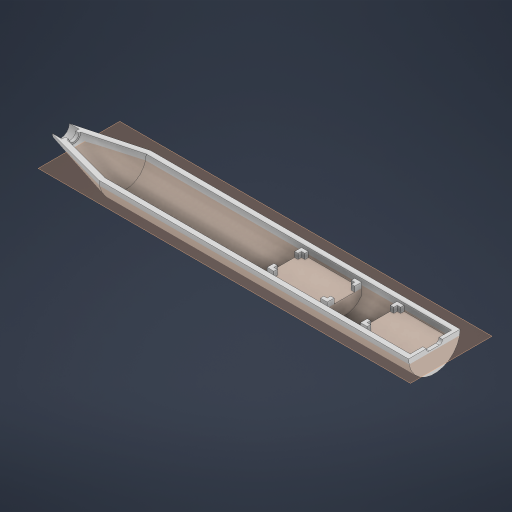
# Autodesk Inventor part: Half bottom
Saved by Autodesk Inventor 2023 (Build 270158000, 158)
## iProperties
Created: 2023-12-06
Part Number: Half bottom
Material: Generic
Document SubType Name: Modeling
Designer: Andi
Density: 1 g/cm^3
Appearance: Default
Author: Andi
Autodesk Inventor part; units mm, degrees
ref_plane "YZ Plane" through (0, 0, 0) normal (1, 0, 0) x (0, 1, 0)
ref_plane "XY Plane" through (0, 0, 0) normal (0, 0, 1) x (1, 0, 0)
sketch "Sketch1" plane through (0, 0, 0) normal (0, 1, 0) x (-1, 0, 0)
  line L0 (90, -15) -> (-90, -15)
  line L1 (-90, -15) -> (-90, 0)
  line L2 (-90, 15) -> (90, 15) construction
  line L3 (90, -15) -> (127.3205, -5)
  line L4 (145.9808, 0) -> (127.3205, 5) construction
  line L5 (127.3205, -5) -> (145.9808, 0) construction
  line L6 (127.3205, 5) -> (90, 15) construction
  line L7 (145.9808, 0) -> (-90, 0)
  line L8 (-88, -12) -> (89.605, -12)
  line L9 (89.605, -12) -> (119.6622, -3.9462)
  line L10 (-90, 0) -> (-88, 0)
  line L11 (-88, 0) -> (-88, -12)
  line L12 (-90, 0) -> (-90, 15) construction
  arc A0 (126.6622, -5) -> (126.6622, 5) centre (126.6622, 0) ccw construction
  line L13 (126.6622, -5) -> (121.6622, -5) construction
  line L14 (121.6622, -5) -> (121.6622, 5) construction
  line L15 (121.6622, 5) -> (126.6622, 5) construction
  line L16 (90, -15) -> (90, 15) construction
  line L17 (119.6622, -3.9462) -> (119.6622, -3)
  line L18 (119.6622, -3) -> (121.6622, -3)
  line L19 (121.6622, -3) -> (121.6622, -5)
  line L20 (121.6622, -5) -> (127.3205, -5)
  point P0 (0, 0)
  point P1 (-88, 0)
  point P2 (131.6622, 0)
  point P3 (90, 0)
  dimension "d0" = 180
  dimension "d1" = 30
  dimension "d2" = 3
  dimension "d3" = 2
  dimension "d5" = 30
  dimension "d6" = 90
  dimension "d9" = 3
  dimension "d24" = 10
  dimension "d25" = 10
  dimension "d26" = 2
  dimension "d29" = 2
  constraints: 43 end point, 8 perpendicular, 3 horizontal, 3 point on circle, 3 tangent, 2 collinear, 2 equal length, 2 horizontal alignment, 2 parallel, 2 point on line, 2 vertical, 1 centre point, 1 midpoint
  measures "d0" distance of L2.start L2.end
  measures "d1" distance of L0.end L2.start
  measures "d2" distance between parallel lines of L8 L0
  measures "d3" distance between parallel lines of L11 L1
  measures "d5" angle of L4 L5
  measures "d6" distance from line of point (0, 0) L1
  measures "d9" distance between parallel lines of L9 L3
  measures "d24" diameter of A0
  measures "d25" distance from line of point (131.662, 0) L14
  measures "d26" distance of L17.end L18.end
  measures "d29" distance of L18.end L13.end
revolve "Revolution1" add sketch "Sketch1" angle 180 about axis through (-145.9808, 0, 0) along (-1, 0, 0)
ref_plane "Work Plane1" through (0, -3, 0) normal (0, 1, 0) x (-1, 0, 0)
sketch "Sketch2" plane through (0, -3, 0) normal (0, 1, 0) x (-1, 0, 0)
  line L0 (-57.7, -10.7) -> (-88, -10.7)
  line L1 (-88, -10.7) -> (-88, 10.7)
  line L2 (-88, 10.7) -> (-57.7, 10.7)
  line L3 (-57.7, 10.7) -> (-57.7, -10.7)
  line L4 (-88, -12) -> (-88, 12) construction
  line L5 (-88, -12) -> (-88, 12) construction
  line L6 (-2.7, -10) -> (-37.7, -10)
  line L7 (-37.7, -10) -> (-37.7, 10)
  line L8 (-37.7, 10) -> (-2.7, 10)
  line L9 (-2.7, 10) -> (-2.7, -10)
  line L10 (17.6, 0) -> (-105.6, 0) construction
  point P0 (0, 0)
  point P1 (-88, 0)
  point P2 (-57.7, 0)
  point P3 (-37.7, 0)
  point P4 (-88, 0)
  point P5 (-88, 0)
  point P6 (-88, 0)
  point P7 (-88, 0)
  point P8 (-59.7, -8.7)
  point P9 (-59.7, 8.7)
  dimension "d20" = 35
  dimension "d21" = 20
  dimension "d39" = 20
  dimension "d42" = 2
  dimension "d43" = 2
  constraints: 16 end point, 7 midpoint, 4 parallel, 2 horizontal, 2 horizontal alignment, 2 perpendicular, 1 point on line, 2 other
  measures "d20" distance of L6.start L6.end
  measures "d21" distance of L8.end L6.start
  measures "d39" distance between parallel lines of L7 L3
  measures "d42" distance from line of point (-59.7, -8.7) L0
  measures "d43" distance from line of L3 point (-59.7, -8.7)
sketch "Sketch3" plane through (90, 0, 15) normal (1, 0, 0) x (0, 0, -1)
  arc A0 (17.89, -1.5) -> (17.89, 1.14) centre (17.89, -0.18) ccw construction
  arc A1 (12.11, 1.14) -> (12.11, -1.5) centre (12.11, -0.18) ccw construction
  line L0 (17.89, -0.18) -> (12.11, -0.18) construction
  line L1 (17.89, -2) -> (12.11, -2)
  line L2 (12.11, 1.64) -> (17.89, 1.64)
  arc A2 (17.89, -2) -> (17.89, 1.64) centre (17.89, -0.18) ccw
  arc A3 (12.11, 1.64) -> (12.11, -2) centre (12.11, -0.18) ccw
  point P0 (15, 0)
  point P1 (15, -0.18)
  dimension "d44" = 0.5
  constraints: 8 end point, 4 point on circle, 4 tangent, 2 centre point, 1 horizontal, 1 midpoint, 1 parallel
  measures "d44" radial gap between concentric circles of A0 A2
extrude "Extrusion2" cut sketch "Sketch3" against normal blind 10
extrude "Extrusion3" add sketch "Sketch2" against normal up to surface round surface about axis through (-0.8025, 0, 0) along (-1, 0, 0) radius 12 far side no
sketch "Sketch4" plane through (0, -3, 0) normal (0, 1, 0) x (1, 0, 0)
  line L0 (57.7, 10.7) -> (61.7, 10.7)
  line L1 (57.7, 10.7) -> (88, 10.7) projected
  line L2 (61.7, 8.7) -> (61.7, 10.7)
  line L3 (61.7, 8.7) -> (59.7, 8.7)
  line L4 (59.7, 8.7) -> (59.7, 6.7)
  line L5 (59.7, 6.7) -> (57.7, 6.7)
  line L6 (57.7, 6.7) -> (57.7, 10.7)
  line L7 (2.7, 10) -> (6.7, 10)
  line L8 (6.7, 10) -> (6.7, 8)
  line L9 (6.7, 8) -> (4.7, 8)
  line L10 (4.7, 8) -> (4.7, 6)
  line L11 (4.7, 6) -> (2.7, 6)
  line L12 (2.7, 6) -> (2.7, 10)
  line L13 (33.7, 10) -> (33.7, 8)
  line L14 (33.7, 8) -> (35.7, 8)
  line L15 (33.7, 10) -> (37.7, 10)
  line L16 (37.7, 10) -> (37.7, 6)
  line L17 (37.7, 6) -> (35.7, 6)
  line L18 (35.7, 6) -> (35.7, 8)
  point P0 (0, 0)
  point P1 (57.7, -10.7)
  point P2 (59.7, -8.7)
  point P3 (2.7, 10)
  point P4 (37.7, 10)
  dimension "d45" = 4
  dimension "d48" = 2
  dimension "d49" = 4
  constraints: 36 end point, 12 perpendicular, 7 equal length, 4 horizontal, 2 coincident, 2 point on line, 1 horizontal alignment, 1 parallel, 2 other
  measures "d45" distance of L5.end L0.start
  measures "d48" distance of L16.end L17.end
  measures "d49" distance of L15.end L16.end
extrude "Extrusion4" add sketch "Sketch4" along normal blind 3
mirror "Mirror1" about plane through (0, 0, 0) normal (0, 0, 1) of "Extrusion4"
equation "\"d9\" = d2"
body "Solid1"
